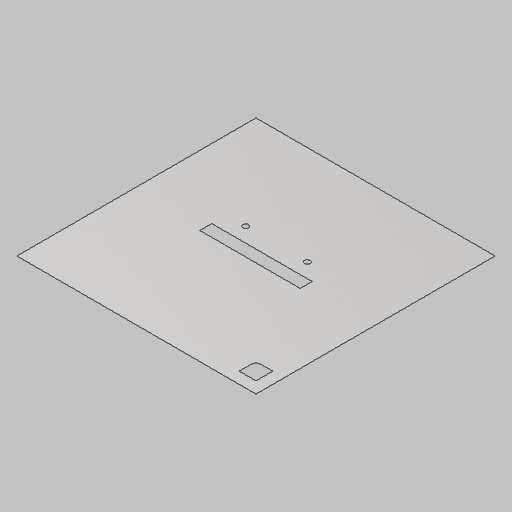
# Autodesk Inventor part: Chapa - aço galvanizado
Saved by Autodesk Inventor 2025.2 (Build 292293000, 293)
## iProperties
Created: 2024-04-26
Part Number: Chapa - aço galvanizado
Material: Genérico
Document SubType Name: Modeling
Designer: phmca
Density: 1 g/cm^3
Appearance: Refletiva cinza claro
Author: phmca
Autodesk Inventor part; units mm, degrees
ref_plane "YZ Plane" through (0, 0, 0) normal (1, 0, 0) x (0, 1, 0)
ref_plane "XZ Plane" through (0, 0, 0) normal (0, 1, 0) x (-1, 0, 0)
ref_plane "XY Plane" through (0, 0, 0) normal (0, 0, 1) x (1, 0, 0)
sketch "Esboço1" plane through (0, 0, 0) normal (0, 1, 0) x (-1, 0, 0)
  line L0 (-250, 250) -> (250, 250)
  line L1 (250, 250) -> (250, -250)
  line L2 (250, -250) -> (-250, -250)
  line L3 (-250, -250) -> (-250, 250)
  line L4 (-250, 250) -> (250, -250) construction
  line L5 (250, 250) -> (-250, -250) construction
  point P0 (0, 0)
  dimension "d0" = 500
  dimension "d1" = 500
  constraints: 12 end point, 2 midpoint, 2 parallel, 1 horizontal, 1 perpendicular
  measures "d0" distance of L1.end L2.end
  measures "d1" distance of L0.end L1.end
extrude "Extrusão1" add sketch "Esboço1" along normal mid plane 1
sketch "Esboço2" plane through (0, 0.5, 0) normal (0, 1, 0) x (1, 0, 0)
  line L0 (-105, -12.5) -> (105, -12.5)
  line L1 (105, -12.5) -> (105, 12.5)
  line L2 (105, 12.5) -> (-105, 12.5)
  line L3 (-105, 12.5) -> (-105, -12.5)
  line L4 (-105, -12.5) -> (105, 12.5) construction
  line L5 (105, -12.5) -> (-105, 12.5) construction
  point P0 (0, 0)
  dimension "d4" = 210
  dimension "d5" = 25
  constraints: 12 end point, 2 midpoint, 2 parallel, 1 horizontal, 1 perpendicular
  measures "d4" distance of L2.end L1.end
  measures "d5" distance of L1.end L0.end
extrude "Extrusão2" cut sketch "Esboço2" along normal mid plane 42.75
sketch "Esboço6" plane through (0, 0.5, 0) normal (0, 1, 0) x (1, 0, 0)
  circle A0 centre (-64.5, 43) radius 6
  circle A1 centre (64.5, 43) radius 6
  line L0 (250, 250) -> (-250, 250) projected
  line L1 (-250, 250) -> (-250, -250) projected
  line L2 (-64.5, 43) -> (64.5, 43) construction
  line L3 (226, -226) -> (191, -226)
  line L4 (191, -226) -> (191, -201)
  line L5 (201, -191) -> (226, -191)
  line L6 (226, -191) -> (226, -226)
  line L7 (250, -250) -> (250, 250) projected
  line L8 (-250, -250) -> (250, -250) projected
  arc A2 (201, -191) -> (191, -201) centre (201, -201) ccw
  point P0 (0, 0)
  point P1 (191, -191)
  dimension "d33" = 12
  dimension "d34" = 12
  dimension "d35" = 207
  dimension "d36" = 185.5
  dimension "d37" = 129
  dimension "d38" = 35
  dimension "d39" = 35
  dimension "d40" = 24
  dimension "d41" = 24
  dimension "d42" = 10
  constraints: 10 end point, 3 centre point, 2 horizontal, 2 parallel, 2 point on circle, 2 point on line, 2 tangent, 1 perpendicular
  measures "d33" diameter of A0
  measures "d34" diameter of A1
  measures "d35" distance from line of L0 L2.start
  measures "d36" distance from line of L1 L2.start
  measures "d37" distance of L2.start L2.end
  measures "d38" distance of point (191, -191) L5.end
  measures "d39" distance of L3.end point (191, -191)
  measures "d40" distance between parallel lines of L7 L6
  measures "d41" distance between parallel lines of L8 L3
  measures "d42" radius of A2
extrude "Extrusão3" cut sketch "Esboço6" against normal up to surface (1 mm away) contours A0 | A1 | L3 L4 A2 L5 L6
